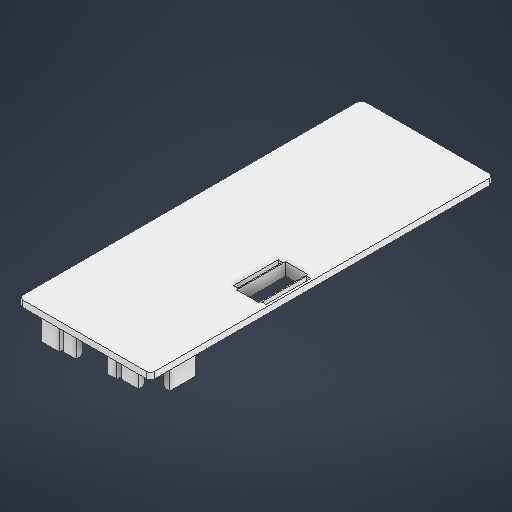
# Autodesk Inventor part: module-lid_command
Saved by Autodesk Inventor 2025.4 (Build 294407000, 407)
## iProperties
Created: 2025-09-05
Part Number: module-lid_command
Material: PC/ABS Plastic
Document SubType Name: Modeling
Designer: sam
Density: 1.1 g/cm^3
Appearance: Smooth - White
Author: sam
Autodesk Inventor part; units mm, degrees
ref_plane "YZ Plane" through (0, 0, 0) normal (1, 0, 0) x (0, 1, 0)
ref_plane "XZ Plane" through (0, 0, 0) normal (0, 1, 0) x (-1, 0, 0)
ref_plane "XY Plane" through (0, 0, 0) normal (0, 0, 1) x (1, 0, 0)
sketch "Sketch1" plane through (0, 0, 0) normal (0, 1, 0) x (-1, 0, 0)
  line L0 (-31.2, -81) -> (31.2, -81)
  line L1 (31.2, -81) -> (31.2, 81)
  line L2 (31.2, 81) -> (-31.2, 81)
  line L3 (-31.2, 81) -> (-31.2, -81)
  line L4 (-31.2, -81) -> (31.2, 81) construction
  line L5 (31.2, -81) -> (-31.2, 81) construction
  point P0 (0, 0)
  dimension "d0" = 62.4
  dimension "d1" = 162
  constraints: 12 end point, 2 midpoint, 2 parallel, 1 horizontal, 1 perpendicular
  measures "d0" distance of L2.end L1.end
  measures "d1" distance of L1.end L0.end
extrude "Extrusion1" add sketch "Sketch1" against normal blind 3
sketch "Sketch2" plane through (0, -3, 0) normal (0, -1, 0) x (1, 0, 0)
  line L0 (-31.2, 81) -> (-31.2, -81) projected
  line L1 (-31.2, -81) -> (31.2, -81) projected
  line L2 (31.2, -81) -> (31.2, 81) projected
  line L3 (31.2, 81) -> (-31.2, 81) projected
  line L4 (28, 77.8) -> (-28, 77.8)
  line L5 (-28, 77.8) -> (-28, -77.8)
  line L6 (-28, -77.8) -> (28, -77.8)
  line L7 (28, -77.8) -> (28, 77.8)
  line L8 (28, 77.8) -> (-28, -77.8) construction
  line L9 (-28, 77.8) -> (28, -77.8) construction
  point P0 (0, 0)
  dimension "d4" = 3.2
  dimension "d5" = 3.2
  constraints: 12 end point, 2 midpoint, 2 parallel, 1 horizontal, 1 perpendicular
  measures "d4" distance between parallel lines of L5 L0
  measures "d5" distance between parallel lines of L1 L6
extrude "Extrusion2" add sketch "Sketch2" along normal blind 3 contours L7 L6 L5 L4
fillet "Fillet1" radius 2 8 edges at (28, -4.5, 77.8) (-28, -4.5, 77.8) (31.2, -1.5, 81) (-31.2, -1.5, 81) (28, -4.5, -77.8) (31.2, -1.5, -81) (-28, -4.5, -77.8) (-31.2, -1.5, -81)
fillet "Fillet2" radius 0.5 8 edges at (-27.4142, -6, 77.2142) (-28, -6, 0) (-27.4142, -6, -77.2142) (0, -6, -77.8) (27.4142, -6, -77.2142) (28, -6, 0) (27.4142, -6, 77.2142) (0, -6, 77.8)
sketch "Sketch3" plane through (0, -6, 0) normal (0, -1, 0) x (1, 0, 0)
  line L0 (26, 77.8) -> (-26, 77.8) projected
  arc A0 (-26, 77.8) -> (-28, 75.8) centre (-26, 75.8) ccw projected
  arc A1 (28, 75.8) -> (26, 77.8) centre (26, 75.8) ccw projected
  line L1 (28, -75.8) -> (28, 75.8) projected
  line L2 (-28, 75.8) -> (-28, -75.8) projected
  line L3 (22.2, 77.8) -> (14.14, 77.8)
  line L4 (14.14, 77.8) -> (14.14, 74.8)
  line L5 (14.14, 74.8) -> (22.2, 74.8)
  line L6 (22.2, 74.8) -> (22.2, 77.8)
  line L7 (31.2, -79) -> (31.2, 79) projected
  point P0 (0, 0)
  point P1 (-17.6788, 77.8)
  point P2 (-8.3626, 77.8)
  dimension "d10" = 8.06
  dimension "d11" = 3
  dimension "d18" = 9
  constraints: 8 end point, 3 point on line, 2 parallel, 1 horizontal, 1 perpendicular
  measures "d10" distance of L5.end L4.end
  measures "d11" distance of L4.end L3.end
  measures "d18" distance between parallel lines of L7 L6
extrude "Extrusion3" add sketch "Sketch3" along normal blind 9.3 from surface at -3
sketch "Sketch4" plane through (0, -6, 0) normal (0, -1, 0) x (1, 0, 0)
  line L0 (14.14, 77.8) -> (-26, 77.8) projected
  line L1 (-23.7, 77.8) -> (-15, 77.8)
  line L2 (-15, 77.8) -> (-15, 74.8)
  line L3 (-15, 74.8) -> (-23.7, 74.8)
  line L4 (-23.7, 74.8) -> (-23.7, 77.8)
  line L5 (-31.2, 79) -> (-31.2, -79) projected
  point P0 (0, 0)
  dimension "d19" = 8.7
  dimension "d20" = 3
  dimension "d21" = 7.5
  constraints: 8 end point, 2 parallel, 1 horizontal, 1 perpendicular, 1 point on line
  measures "d19" distance of L2.end L3.end
  measures "d20" distance of L1.end L2.end
  measures "d21" distance between parallel lines of L5 L4
extrude "Extrusion4" add sketch "Sketch4" along normal blind 12.8 from surface at -3
sketch "Sketch5" plane through (0, -6, 0) normal (0, -1, 0) x (1, 0, 0)
  line L0 (-26, 77.8) -> (26, 77.8) projected
  line L1 (-7.15, 77.8) -> (-13.25, 77.8)
  line L2 (-13.25, 77.8) -> (-13.25, 74.8)
  line L3 (-13.25, 74.8) -> (-7.15, 74.8)
  line L4 (-7.15, 74.8) -> (-7.15, 77.8)
  line L5 (31.2, -79) -> (31.2, 79) projected
  line L6 (-31.2, 79) -> (-31.2, -79) projected
  point P0 (0, 0)
  dimension "d24" = 6.1
  dimension "d25" = 3
  dimension "d29" = 17.95
  constraints: 8 end point, 2 parallel, 1 horizontal, 1 perpendicular, 1 point on line
  measures "d24" distance of L3.end L2.end
  measures "d25" distance of L2.end L1.end
  measures "d29" distance between parallel lines of L6 L2
extrude "Extrusion5" add sketch "Sketch5" along normal blind 11.8 from surface at -3
sketch "Sketch6" plane through (0, -6, 0) normal (0, -1, 0) x (1, 0, 0)
  line L0 (28, 75.8) -> (28, -75.8) projected
  line L1 (28, 67.8) -> (24, 67.8)
  line L2 (24, 67.8) -> (24, 55.7)
  line L3 (24, 55.7) -> (28, 55.7)
  line L4 (28, 55.7) -> (28, 67.8)
  line L5 (26, 77.8) -> (22.2, 77.8) projected
  line L6 (28, 55.7) -> (27, 55.7)
  line L7 (27, 55.7) -> (27, 67.8)
  line L8 (27, 67.8) -> (28, 67.8)
  line L9 (28, 67.8) -> (28, 55.7)
  point P0 (0, 0)
  dimension "d33" = 4
  dimension "d34" = 12.1
  dimension "d35" = 10
  dimension "d36" = 1
  constraints: 16 end point, 4 parallel, 2 horizontal, 2 perpendicular, 2 point on line
  measures "d33" distance of L3.end L2.end
  measures "d34" distance of L2.end L1.end
  measures "d35" distance between parallel lines of L5 L1
  measures "d36" distance of L7.end L8.end
extrude "Extrusion6" add sketch "Sketch6" along normal blind 12.8 from surface at -3 contours L7 L3 L2 L1
sketch "Sketch9" plane through (0, -6, 0) normal (0, -1, 0) x (1, 0, 0)
  line L0 (14.14, 77.8) -> (-7.15, 77.8) projected
  line L1 (12.14, 77.8) -> (7.44, 77.8)
  line L2 (7.44, 77.8) -> (7.44, 74.8)
  line L3 (7.44, 74.8) -> (12.14, 74.8)
  line L4 (12.14, 74.8) -> (12.14, 77.8)
  line L5 (14.14, 74.8) -> (14.14, 77.8) projected
  point P0 (0, 0)
  point P1 (11.14, 72.8)
  dimension "d57" = 4.7
  dimension "d58" = 3
  dimension "d59" = 2
  constraints: 8 end point, 2 parallel, 1 horizontal, 1 perpendicular, 1 point on line, 1 other
  measures "d57" distance of L3.end L2.end
  measures "d58" distance of L2.end L1.end
extrude "Extrusion9" add sketch "Sketch9" along normal blind 10.4 from surface at -3
sketch "Sketch7" plane through (0, 0, 0) normal (0, 1, 0) x (1, 0, 0)
  line L0 (17.2, -3.2) -> (27.6, -3.2)
  line L1 (27.6, -3.2) -> (27.6, -26.3)
  line L2 (27.6, -26.3) -> (17.2, -26.3)
  line L3 (17.2, -26.3) -> (17.2, -3.2)
  line L4 (-29.2, -81) -> (29.2, -81) projected
  line L5 (31.2, -79) -> (31.2, 79) projected
  point P0 (0, 0)
  dimension "d39" = 10.4
  dimension "d40" = 23.1
  dimension "d43" = 54.7
  dimension "d44" = 3.6
  constraints: 8 end point, 2 parallel, 1 horizontal, 1 perpendicular
  measures "d39" distance of L1.end L2.end
  measures "d40" distance of L0.end L1.end
  measures "d43" distance between parallel lines of L4 L2
  measures "d44" distance between parallel lines of L5 L1
extrude "Extrusion7" cut sketch "Sketch7" against normal through all
sketch "Sketch8" plane through (0, 0, 0) normal (0, 1, 0) x (1, 0, 0)
  line L0 (27.6, -3.2) -> (27.6, -26.3) projected
  line L1 (27.6, -26.3) -> (17.2, -26.3) projected
  line L2 (17.2, -26.3) -> (17.2, -3.2) projected
  line L3 (17.2, -3.2) -> (27.6, -3.2) projected
  arc A0 (-29.2, 81) -> (-31.2, 79) centre (-29.2, 79) ccw projected
  line L4 (-31.2, 79) -> (-31.2, -79) projected
  arc A1 (-31.2, -79) -> (-29.2, -81) centre (-29.2, -79) ccw projected
  line L5 (-29.2, -81) -> (29.2, -81) projected
  arc A2 (29.2, -81) -> (31.2, -79) centre (29.2, -79) ccw projected
  line L6 (31.2, -79) -> (31.2, 79) projected
  arc A3 (31.2, 79) -> (29.2, 81) centre (29.2, 79) ccw projected
  line L7 (29.2, 81) -> (-29.2, 81) projected
  line L8 (16.7, -4.2) -> (14.7, -4.2)
  line L9 (14.7, -4.2) -> (14.7, -25.3)
  line L10 (14.7, -25.3) -> (16.7, -25.3)
  line L11 (16.7, -25.3) -> (16.7, -4.2)
  line L12 (28.1, -4.2) -> (30.1, -4.2)
  line L13 (30.1, -4.2) -> (30.1, -25.3)
  line L14 (30.1, -25.3) -> (28.1, -25.3)
  line L15 (28.1, -25.3) -> (28.1, -4.2)
  point P0 (0, 0)
  dimension "d45" = 2
  dimension "d48" = 2
  dimension "d49" = 1
  dimension "d50" = 1
  dimension "d51" = 1
  dimension "d52" = 1
  dimension "d53" = 0.5
  dimension "d54" = 0.5
  constraints: 16 end point, 4 parallel, 2 horizontal, 2 perpendicular
  measures "d45" distance of L10.end L9.end
  measures "d48" distance of L13.end L14.end
  measures "d49" distance between parallel lines of L3 L8
  measures "d50" distance between parallel lines of L1 L10
  measures "d51" distance between parallel lines of L14 L1
  measures "d52" distance between parallel lines of L3 L12
  measures "d53" distance between parallel lines of L2 L11
  measures "d54" distance between parallel lines of L15 L0
extrude "Extrusion8" cut sketch "Sketch8" against normal blind 2 contours L11 L10 L9 L8 | L12 L13 L14 L15
chamfer "Chamfer2" distance 1 angle 45 5 edges at (-19.35, -15.8, 74.8) (-10.2, -14.8, 74.8) (9.79, -13.4, 74.8) (18.17, -12.3, 74.8) (24, -15.8, 61.75)
body "Solid1"
